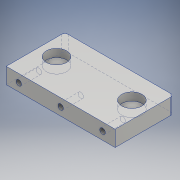
# Autodesk Inventor part: suporte_guia_linear_cabeça_superior
Saved by Autodesk Inventor 2018 (Build 220112000, 112)
## iProperties
Created: 2018-05-17
Part Number: suporte_guia_linear_cabeça_superior
Material: Alumínio 6061
Document SubType Name: Modeling
Designer: Usuario
Density: 2.7 g/cm^3
Appearance: Alumínio - Plano
Author: Usuario
Autodesk Inventor part; units mm, degrees
ref_plane "YZ Plane" through (0, 0, 0) normal (1, 0, 0) x (0, 1, 0)
ref_plane "XZ Plane" through (0, 0, 0) normal (0, 1, 0) x (-1, 0, 0)
ref_plane "XY Plane" through (0, 0, 0) normal (0, 0, 1) x (1, 0, 0)
sketch "Esboço12" plane through (0, 0, 0) normal (0, 0, 1) x (1, 0, 0)
  line L0 (0, 0) -> (-32.5, 0)
  line L1 (-32.5, 0) -> (-32.5, 33)
  line L2 (-30.5, 35) -> (0, 35)
  line L3 (0, 44.9607) -> (0, -19.7308) construction
  circle A0 centre (-22.5, 22) radius 6 construction
  arc A1 (-30.5, 35) -> (-32.5, 33) centre (-30.5, 33) ccw
  circle A2 centre (-22.5, 22) radius 6 construction
  line L4 (0, 0) -> (32.5, 0)
  line L5 (32.5, 0) -> (32.5, 33)
  line L6 (30.5, 35) -> (0, 35)
  circle A3 centre (22.5, 22) radius 6 construction
  arc A4 (32.5, 33) -> (30.5, 35) centre (30.5, 33) ccw
  circle A5 centre (22.5, 22) radius 6 construction
  point P0 (-32.5, 35)
  point P1 (32.5, 35)
  dimension "d95" = 32.5
  dimension "d96" = 35
  dimension "d97" = 2
  dimension "d99" = 13
  dimension "d100" = 10
  constraints: 14 end point, 7 symmetric about line, 6 centre point, 4 point on circle, 4 point on line, 2 coincident, 2 perpendicular, 2 tangent, 1 horizontal, 1 vertical, 3 other
  measures "d95" distance of L0.start L0.end
  measures "d96" distance of L0.end point (-32.5, 35)
  measures "d97" radius of A1
  measures "d99" distance from line of L2 A0.centre
  measures "d100" distance from line of L1 A0.centre
extrude "Extrusão2" add sketch "Esboço12" along normal mid plane 9.5
sketch "Esboço13" plane through (0, 0, 4.75) normal (0, 0, 1) x (1, 0, 0)
  circle A0 centre (-22.5, 20) radius 6 construction
  line L0 (-32.5, 33) -> (-32.5, 0) projected
  line L1 (30.5, 35) -> (-30.5, 35) projected
  line L2 (0, 35) -> (0, 0) construction
  circle A1 centre (22.5, 20) radius 6 construction
  dimension "d103" = 12
  dimension "d104" = 10
  dimension "d105" = 15
  constraints: 2 centre point, 2 end point, 1 midpoint, 1 symmetric about line, 1 vertical, 1 other
  measures "d103" diameter of A0
  measures "d104" distance from line of A0.centre L0
  measures "d105" distance from line of A0.centre L1
hole "Furo7" at (-22.5, 20, 4.75) at (22.5, 20, 4.75) direction (0, 0, -1) diameter 12.1 depth 4.75
sketch "Esboço14" plane through (-32.5, 0, 4.75) normal (0, -1, 0) x (1, 0, 0)
  line L0 (32.5, -4.75) -> (0, -4.75) construction
  line L1 (32.5, -4.75) -> (65, -4.75) construction
  line L2 (61.05, -4.75) -> (48.95, -4.75) construction
  circle A0 centre (32.5, -4.75) radius 2 construction
  circle A1 centre (7.5, -4.75) radius 2 construction
  circle A2 centre (57.5, -4.75) radius 2 construction
  circle A3 centre (32.5, -4.75) radius 2 construction
  dimension "d113" = 32.5
  dimension "d114" = 32.5
  dimension "d115" = 4
  dimension "d118" = 25
  dimension "d121" = 25
  constraints: 4 centre point, 4 end point, 3 horizontal, 1 coincident, 1 collinear, 6 other
  measures "d113" distance of L0.start L0.end
  measures "d114" distance of L0.start L1.end
  measures "d115" diameter of A0
  measures "d118" distance of A0.centre A1.centre
  measures "d121" distance of A0.centre A2.centre
hole "Furo8" at (-25, 0, 0) at (0, 0, 0) at (25, 0, 0) direction (0, 1, 0) diameter 3.242 depth 12 thread size "M4x0.7" class "6H" standard "ANSI Metric M Profile"
